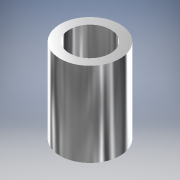
# Autodesk Inventor part: Parts_MetalCollar_Ph2_L4.5
Saved by Autodesk Inventor 2018.2 (Build 222227000, 227)
## iProperties
Created: 2015-02-23
Part Number: Parts_MetalCollar_Ph2_L4.5
Material: ステンレス鋼
Document SubType Name: Modeling
Designer: Yamaura
Density: 8 g/cm^3
Appearance: アルミニウム - フラット
Catalog Web Link: http://wilco.jp/products/U/CU-PH.html
Description: CU-2004.5PH
Vendor: wilco
Author: Yamaura
Title: Parts_MetalCollar_Ph2_L4.5
Autodesk Inventor part; units mm, degrees
ref_plane "YZ Plane" through (0, 0, 0) normal (1, 0, 0) x (0, 1, 0)
ref_plane "XZ Plane" through (0, 0, 0) normal (0, 1, 0) x (-1, 0, 0)
ref_plane "XY Plane" through (0, 0, 0) normal (0, 0, 1) x (1, 0, 0)
sketch "スケッチ1" plane through (0, 0, 0) normal (1, 0, 0) x (0, 1, 0)
  line L0 (1.1, 0) -> (1.6, 0)
  line L1 (1.6, 0) -> (1.6, -4.5)
  line L2 (1.6, -4.5) -> (1.1, -4.5)
  line L3 (1.1, -4.5) -> (1.1, 0)
  line L4 (0, -5.4) -> (0, 0.9) projected
  point P0 (0, 0)
  dimension "d0" = 1.1
  dimension "d1" = 1.6
  dimension "d2" = 4.5
  constraints: 8 end point, 2 parallel, 1 horizontal, 1 perpendicular, 1 point on line
  measures "d0" distance from line of L3 point (0, 0)
  measures "d1" distance from line of L1 point (0, 0)
  measures "d2" distance of L0.end L1.end
revolve "回転1" add sketch "スケッチ1" angle 360 about axis through (0, 0, -10) along (0, 0, 1)
